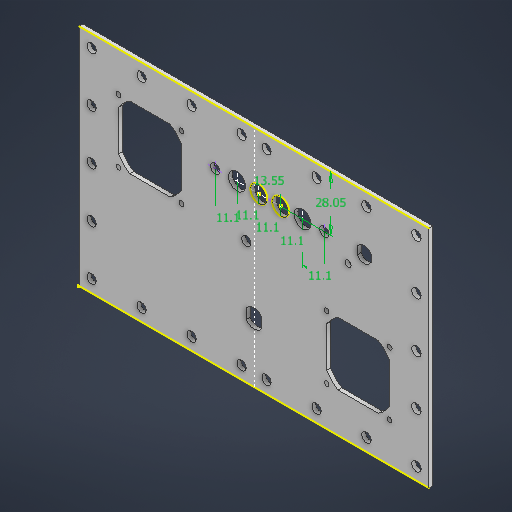
# Autodesk Inventor part: NRDZ_Fan_plate
Saved by Autodesk Inventor 2026.2 (Build 302298010, 298A)
## iProperties
Created: 2026-06-10
Part Number: NRDZ_Fan_plate
Material: Generic
Document SubType Name: Modeling
Designer: sonata
Density: 1 g/cm^3
Appearance: Default
Author: sonata
Autodesk Inventor part; units mm, degrees
ref_plane "YZ Plane" through (0, 0, 0) normal (1, 0, 0) x (0, 1, 0)
ref_plane "XZ Plane" through (0, 0, 0) normal (0, 1, 0) x (-1, 0, 0)
ref_plane "XY Plane" through (0, 0, 0) normal (0, 0, 1) x (1, 0, 0)
sketch "Sketch1" plane through (0, 0, 0) normal (0, 0, 1) x (1, 0, 0)
  line L0 (0, 0) -> (177.8, 0)
  line L1 (177.8, 0) -> (177.8, 114.3)
  line L2 (177.8, 114.3) -> (0, 114.3)
  line L3 (0, 114.3) -> (0, 0)
  dimension "d0" = 177.8
  dimension "d1" = 114.3
  constraints: 8 end point, 2 parallel, 1 horizontal, 1 perpendicular
  measures "d0" distance of L1.end L2.end
  measures "d1" distance of L0.end L1.end
extrude "Extrusion1" add sketch "Sketch1" along normal blind 2
sketch "Sketch2" plane through (0, 0, 2) normal (0, 0, 1) x (1, 0, 0)
  line L0 (0, 114.3) -> (0, 0) projected
  line L1 (177.8, 114.3) -> (0, 114.3) projected
  line L2 (177.8, 0) -> (177.8, 114.3) projected
  point P0 (6.35, 107.95)
  point P1 (6.35, 82.55)
  point P2 (6.35, 57.15)
  point P3 (6.35, 31.75)
  point P4 (6.35, 6.35)
  point P5 (31.75, 6.35)
  point P6 (57.15, 6.35)
  point P7 (82.55, 6.35)
  point P8 (95.25, 6.35)
  point P9 (146.05, 6.35)
  point P10 (120.65, 6.35)
  point P11 (171.45, 6.35)
  point P12 (171.45, 31.75)
  point P13 (171.45, 57.15)
  point P14 (171.45, 82.55)
  point P15 (171.45, 107.95)
  point P16 (120.65, 107.95)
  point P17 (146.05, 107.95)
  point P18 (95.25, 107.95)
  point P19 (82.55, 107.95)
  point P20 (57.15, 107.95)
  point P21 (31.75, 107.95)
  dimension "d4" = 25.4
  dimension "d5" = 6.35
  dimension "d7" = 6.35
  dimension "d8" = 25.4
  dimension "d9" = 25.4
  dimension "d10" = 25.4
  dimension "d11" = 25.4
  dimension "d12" = 25.4
  dimension "d13" = 25.4
  dimension "d14" = 6.35
  dimension "d15" = 25.4
  dimension "d16" = 25.4
  dimension "d17" = 25.4
  constraints: 17 horizontal alignment, 14 vertical alignment
  measures "d4" distance of point (31.75, 107.95) point (6.35, 107.95)
  measures "d5" distance from line of L0 point (6.35, 107.95)
  measures "d7" distance from line of point (6.35, 107.95) L1
  measures "d8" distance of point (6.35, 82.55) point (6.35, 107.95)
  measures "d9" distance of point (6.35, 82.55) point (6.35, 57.15)
  measures "d10" distance of point (6.35, 57.15) point (6.35, 31.75)
  measures "d11" distance of point (6.35, 31.75) point (6.35, 6.35)
  measures "d12" distance of point (57.15, 107.95) point (31.75, 107.95)
  measures "d13" distance of point (82.55, 107.95) point (57.15, 107.95)
  measures "d14" distance from line of L2 point (171.45, 107.95)
  measures "d15" distance of point (171.45, 107.95) point (146.05, 107.95)
  measures "d16" distance of point (146.05, 107.95) point (120.65, 107.95)
  measures "d17" distance of point (120.65, 107.95) point (95.25, 107.95)
hole "Hole1" at (6.35, 107.95, 2) at (6.35, 82.55, 2) at (6.35, 57.15, 2) at (6.35, 31.75, 2) at (6.35, 6.35, 2) at (31.75, 6.35, 2) at (57.15, 6.35, 2) at (82.55, 6.35, 2) at (95.25, 6.35, 2) at (146.05, 6.35, 2) at (120.65, 6.35, 2) at (171.45, 6.35, 2) at (171.45, 31.75, 2) at (171.45, 57.15, 2) at (171.45, 82.55, 2) at (171.45, 107.95, 2) at (120.65, 107.95, 2) at (146.05, 107.95, 2) at (95.25, 107.95, 2) at (82.55, 107.95, 2) at (57.15, 107.95, 2) at (31.75, 107.95, 2) direction (0, 0, -1) diameter 4.76 end through all
sketch "Sketch3" plane through (0, 0, 2) normal (0, 0, 1) x (1, 0, 0)
  line L0 (177.8, 114.3) -> (0, 114.3) projected
  line L1 (88.9, 114.3) -> (88.9, 0) construction
  line L2 (0, 0) -> (177.8, 0) projected
  point P0 (91.35, 86.25)
  point P1 (102.45, 86.25)
  point P2 (113.55, 86.25)
  point P3 (80.25, 86.25)
  point P4 (69.15, 86.25)
  point P5 (124.65, 86.25)
  dimension "d25" = 28.05
  dimension "d26" = 13.55
  dimension "d27" = 11.1
  dimension "d28" = 11.1
  dimension "d29" = 11.1
  dimension "d37" = 11.1
  dimension "d38" = 11.1
  constraints: 3 horizontal alignment, 2 end point, 2 midpoint, 1 vertical
  measures "d25" distance from line of L0 point (102.45, 86.25)
  measures "d26" distance from line of L1 point (102.45, 86.25)
  measures "d27" distance of point (102.45, 86.25) point (91.35, 86.25)
  measures "d28" distance of point (113.55, 86.25) point (102.45, 86.25)
  measures "d29" distance of point (91.35, 86.25) point (80.25, 86.25)
  measures "d37" distance of point (80.25, 86.25) point (69.15, 86.25)
  measures "d38" distance of point (124.65, 86.25) point (113.55, 86.25)
hole "Hole2" at (91.35, 86.25, 2) at (102.45, 86.25, 2) at (113.55, 86.25, 2) at (80.25, 86.25, 2) direction (0, 0, -1) diameter 8.7 end through all
hole "Hole3" at (124.65, 86.25, 2) at (69.15, 86.25, 2) direction (0, 0, -1) diameter 4.76 end through all
sketch "Sketch5" plane through (0, 0, 2) normal (0, 0, 1) x (1, 0, 0)
  line L0 (177.8, 114.3) -> (0, 114.3) projected
  line L1 (88.9, 114.3) -> (88.9, 0) construction
  circle A0 centre (88.9, 30.2) radius 4.7
  line L2 (84.95, 27.6529) -> (84.95, 32.7471)
  line L3 (92.85, 27.6529) -> (92.85, 32.7471)
  line L4 (0, 0) -> (177.8, 0) projected
  point P0 (88.9, 0)
  dimension "d46" = 9.4
  dimension "d47" = 7.9
  dimension "d48" = 3.95
  dimension "d49" = 30.2
  constraints: 6 end point, 4 midpoint, 4 point on circle, 2 parallel, 1 centre point, 1 point on line, 1 vertical
  measures "d46" diameter of A0
  measures "d47" distance between parallel lines of L3 L2
  measures "d48" distance between parallel lines of L1 L2
  measures "d49" distance from line of L4 A0.centre
extrude "Extrusion2" cut sketch "Sketch5" against normal through all contours L3 A0 L2
sketch "Sketch6" plane through (0, 0, 2) normal (0, 0, 1) x (1, 0, 0)
  circle A0 centre (144.8, 86.3) radius 4
  line L0 (177.8, 114.3) -> (0, 114.3) projected
  line L1 (177.8, 0) -> (177.8, 114.3) projected
  line L2 (141.3, 84.3635) -> (141.3, 88.2365)
  line L3 (144.8, 86.3) -> (136.6683, 78.1683)
  line L4 (144.8, 86.3) -> (144.8, 114.3)
  circle A1 centre (136.6683, 78.1683) radius 1.6
  point P0 (0, 0)
  dimension "d52" = 28
  dimension "d53" = 33
  dimension "d54" = 8
  dimension "d55" = 7.5
  dimension "d58" = 135
  dimension "d59" = 11.5
  dimension "d60" = 3.2
  constraints: 6 end point, 2 centre point, 2 point on circle, 1 coincident, 1 perpendicular, 1 point on line, 1 vertical
  measures "d52" distance from line of L0 L3.start
  measures "d53" distance from line of L1 L3.start
  measures "d54" diameter of A0
  measures "d58" angle of L4 L3
  measures "d59" distance of L3.start L3.end
  measures "d60" diameter of A1
extrude "Extrusion3" cut sketch "Sketch6" against normal through all contours A0 L4 L3 L2 | A0 L3 L4 | A1
sketch "Sketch7" plane through (0, 0, 2) normal (0, 0, 1) x (1, 0, 0)
  line L0 (177.8, 0) -> (177.8, 114.3) projected
  line L1 (0, 0) -> (177.8, 0) projected
  point P0 (125.8, 52)
  point P1 (157.8, 52)
  point P2 (157.8, 20)
  point P3 (125.8, 20)
  dimension "d61" = 20
  dimension "d62" = 32
  dimension "d63" = 32
  dimension "d64" = 20
  constraints: 2 horizontal alignment, 2 vertical alignment
  measures "d61" distance from line of L0 point (157.8, 52)
  measures "d62" distance of point (125.8, 52) point (157.8, 52)
  measures "d63" distance of point (125.8, 20) point (125.8, 52)
  measures "d64" distance from line of point (157.8, 20) L1
hole "Hole4" at (125.8, 52, 2) at (157.8, 52, 2) at (157.8, 20, 2) at (125.8, 20, 2) direction (0, 0, -1) diameter 2.459 end through all thread size "M3x0.5" class "6H" standard "ANSI Metric M Profile"
sketch "Sketch8" plane through (0, 0, 2) normal (0, 0, 1) x (1, 0, 0)
  line L0 (177.8, 114.3) -> (0, 114.3) projected
  line L1 (0, 114.3) -> (0, 0) projected
  point P0 (20, 94.3)
  point P1 (52, 94.3)
  point P2 (52, 62.3)
  point P3 (20, 62.3)
  dimension "d72" = 32
  dimension "d73" = 32
  dimension "d74" = 20
  dimension "d75" = 20
  constraints: 2 horizontal alignment, 2 vertical alignment
  measures "d72" distance of point (52, 94.3) point (20, 94.3)
  measures "d73" distance of point (52, 62.3) point (52, 94.3)
  measures "d74" distance from line of L0 point (20, 94.3)
  measures "d75" distance from line of point (20, 94.3) L1
hole "Hole5" at (20, 94.3, 2) at (52, 94.3, 2) at (52, 62.3, 2) at (20, 62.3, 2) direction (0, 0, -1) diameter 2.459 end through all thread size "M3x0.5" class "6H" standard "ANSI Metric M Profile"
sketch "Sketch9" plane through (0, 0, 2) normal (0, 0, 1) x (1, 0, 0)
  line L0 (0, 114.3) -> (0, 0) projected
  line L1 (177.8, 114.3) -> (0, 114.3) projected
  point P0 (85, 62.3)
  dimension "d83" = 85
  dimension "d84" = 52
  measures "d83" distance from line of L0 point (85, 62.3)
  measures "d84" distance from line of L1 point (85, 62.3)
hole "Hole6" at (85, 62.3, 2) direction (0, 0, -1) diameter 4.76 end through all
sketch "Sketch10" plane through (0, 0, 2) normal (0, 0, 1) x (1, 0, 0)
  circle A0 centre (20, 94.3) radius 1.2295 projected
  circle A1 centre (52, 94.3) radius 1.2295 projected
  circle A2 centre (52, 62.3) radius 1.2295 projected
  line L0 (20, 94.3) -> (52, 62.3)
  circle A3 centre (20, 62.3) radius 1.2295 projected
  line L1 (20, 62.3) -> (52, 94.3)
  circle A4 centre (36, 78.3) radius 19
  line L2 (20, 62.3) -> (20, 94.3)
  line L3 (20, 94.3) -> (52, 94.3)
  line L4 (52, 94.3) -> (52, 62.3)
  line L5 (20, 62.3) -> (52, 62.3)
  circle A5 centre (125.8, 52) radius 1.2295 projected
  circle A6 centre (157.8, 20) radius 1.2295 projected
  line L6 (125.8, 52) -> (157.8, 20)
  line L7 (157.8, 20) -> (157.8, 52)
  line L8 (157.8, 52) -> (125.8, 52)
  circle A7 centre (125.8, 20) radius 1.2295 projected
  line L9 (125.8, 20) -> (125.8, 52)
  line L10 (125.8, 20) -> (157.8, 52)
  line L11 (157.8, 20) -> (125.8, 20)
  circle A8 centre (141.8, 36) radius 19
  point P0 (0, 0)
  point P1 (125.8, 46.247)
  point P2 (125.8, 25.753)
  point P3 (131.553, 20)
  point P4 (152.047, 20)
  point P5 (157.8, 25.753)
  point P6 (157.8, 46.247)
  point P7 (152.047, 52)
  point P8 (131.553, 52)
  point P9 (20, 88.547)
  point P10 (20, 68.053)
  point P11 (25.753, 62.3)
  point P12 (46.247, 62.3)
  point P13 (52, 68.053)
  point P14 (52, 88.547)
  point P15 (46.247, 94.3)
  point P16 (25.753, 94.3)
  dimension "d92" = 38
  dimension "d93" = 38
  constraints: 24 end point, 6 perpendicular, 2 centre point, 2 midpoint, 2 vertical
  measures "d92" diameter of A4
  measures "d93" diameter of A8
extrude "Extrusion4" cut sketch "Sketch10" against normal blind 10 contours L3 A4 L1 L0 | A4 L0 L1 L2 | L1 A4 L4 L0 | L0 A4 L5 L1 | L8 A8 L10 L6 | A8 L6 L10 L9 | L10 A8 L7 L6 | L6 A8 L11 L10
sketch "Sketch11" plane through (0, 0, 2) normal (0, 0, 1) x (1, 0, 0)
  circle A0 centre (91.35, 86.25) radius 4.35 projected
  line L0 (95.7, 86.25) -> (98.1, 86.25)
  circle A1 centre (102.45, 86.25) radius 4.35 projected
  point P0 (0, 0)
  constraints: 2 end point, 2 horizontal alignment, 1 horizontal, 2 other
body "Solid1"
